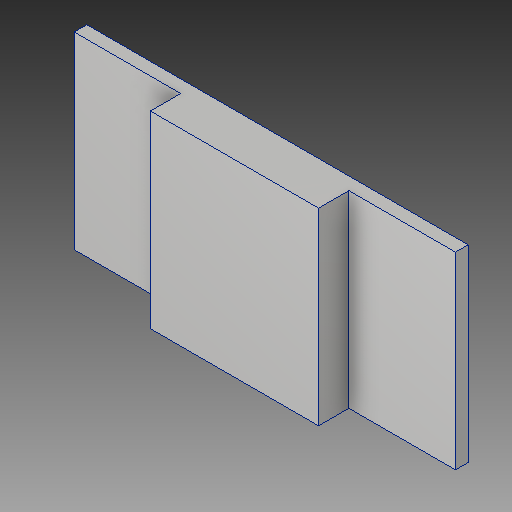
# Autodesk Inventor part: bagcimspacer
Saved by Autodesk Inventor 2017 (Build 210142000, 142)
## iProperties
Created: 2018-02-03
Part Number: bagcimspacer
Material: Aluminum 6061
Document SubType Name: Modeling
Designer: S338674153
Density: 2.7 g/cm^3
Appearance: Aluminum - Flat
Author: S338674153
Autodesk Inventor part; units mm, degrees
ref_plane "YZ Plane" through (0, 0, 0) normal (1, 0, 0) x (0, 1, 0)
ref_plane "XZ Plane" through (0, 0, 0) normal (0, 1, 0) x (-1, 0, 0)
ref_plane "XY Plane" through (0, 0, 0) normal (0, 0, 1) x (1, 0, 0)
sketch "Sketch1" plane through (0, 0, 0) normal (0, 0, 1) x (1, 0, 0)
  line L0 (0, 0) -> (26.6192, 0)
  line L1 (26.6192, 0) -> (26.6192, 47.0916)
  line L2 (26.6192, 47.0916) -> (0, 47.0916)
  line L3 (0, 47.0916) -> (0, 0)
  dimension "d0" = 26.6192
  dimension "d1" = 47.0916
  constraints: 8 end point, 2 parallel, 1 horizontal, 1 perpendicular
  measures "d0" distance of L2.end L1.end
  measures "d1" distance of L1.end L0.end
extrude "Extrusion1" add sketch "Sketch1" along normal blind 3.175
sketch "Sketch6" plane through (26.6192, 0, 0) normal (1, 0, 0) x (0, 0, -1)
  line L0 (0, 0) -> (-10.7442, 0)
  line L1 (-10.7442, 0) -> (-10.7442, 47.0916)
  line L2 (-10.7442, 47.0916) -> (0, 47.0916)
  line L3 (0, 47.0916) -> (0, 0)
  dimension "d15" = 10.7442
  constraints: 8 end point, 2 parallel, 1 horizontal, 1 perpendicular
  measures "d15" distance of L1.end L2.end
extrude "Extrusion6" add sketch "Sketch6" along normal blind 42.0116
sketch "Sketch7" plane through (68.6308, 0, 0) normal (1, 0, 0) x (0, 0, -1)
  line L0 (0, 47.0916) -> (0, 0) projected
  line L1 (-3.175, 47.0916) -> (-3.175, 0) projected
  line L2 (0, 0) -> (-3.175, 0)
  line L3 (-3.175, 0) -> (-3.175, 47.0916)
  line L4 (-3.175, 47.0916) -> (0, 47.0916)
  line L5 (0, 47.0916) -> (0, 0)
  constraints: 8 end point, 2 parallel, 1 horizontal, 1 perpendicular
extrude "Extrusion7" add sketch "Sketch7" along normal blind 26.6192
body "Solid1"
